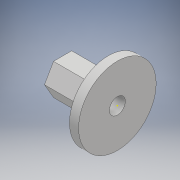
# Autodesk Inventor part: InnerLayerHub3mm
Saved by Autodesk Inventor 2018 (Build 220112000, 112)
## iProperties
Created: 2019-06-05
Part Number: InnerLayerHub3mm
Material: Generic
Document SubType Name: Modeling
Designer: Aditya Kendre
Density: 1 g/cm^3
Appearance: Default
Author: Aditya Kendre
Autodesk Inventor part; units mm, degrees
ref_plane "YZ Plane" through (0, 0, 0) normal (1, 0, 0) x (0, 1, 0)
ref_plane "XZ Plane" through (0, 0, 0) normal (0, 1, 0) x (-1, 0, 0)
ref_plane "XY Plane" through (0, 0, 0) normal (0, 0, 1) x (1, 0, 0)
sketch "Sketch1" plane through (0, 0, 0) normal (1, 0, 0) x (0, 1, 0)
  line L0 (2, 0) -> (-2, 0) construction
  line L1 (-2, 0) -> (-2, -15.7322) construction
  line L2 (-2, -15.7322) -> (2, -15.7322) construction
  line L3 (2, -15.7322) -> (2, 0) construction
  line L4 (2, -3.4446) -> (-1.9831, -3.4544)
  line L5 (-1.9831, -3.4544) -> (-3.9831, -0.0097)
  line L6 (-3.9831, -0.0097) -> (-2, 3.4446)
  line L7 (-2, 3.4446) -> (1.9831, 3.4544)
  line L8 (1.9831, 3.4544) -> (3.9831, 0.0097)
  line L9 (3.9831, 0.0097) -> (2, -3.4446)
  point P0 (0, 0)
  point P1 (0, 0)
  dimension "d0" = 4
  constraints: 20 end point, 2 parallel, 1 coincident, 1 horizontal, 1 perpendicular, 1 point on line, 13 other
  measures "d0" distance of L2.end L1.end
extrude "Extrusion1" add sketch "Sketch1" along normal blind 4 and the other way blind 6
sketch "Sketch2" plane through (4, 0, 0) normal (1, 0, 0) x (0, 0, -1)
  line L0 (3.4446, 2) -> (-0.0097, 3.9831) projected
  circle A0 centre (0, 0) radius 3.9832
  constraints: 1 coincident, 3 other
extrude "Extrusion2" add sketch "Sketch2" along normal blind 2
sketch "Sketch3" plane through (6, 0, 0) normal (1, 0, 0) x (0, 0, -1)
  point P0 (0, 0)
sketch "Sketch4" plane through (4, 0, 0) normal (-1, 0, 0) x (0, 0, 1)
  circle A0 centre (0, 0) radius 6
  dimension "d5" = 12
  constraints: 1 centre point, 1 coincident
  measures "d5" diameter of A0
extrude "Extrusion3" add sketch "Sketch4" against normal blind 2
sketch "Sketch5" plane through (6, 0, 0) normal (1, 0, 0) x (0, 0, -1)
  circle A0 centre (0, 0) radius 1.5
  dimension "d8" = 3
  constraints: 1 centre point, 1 coincident
  measures "d8" diameter of A0
extrude "Extrusion4" cut sketch "Sketch5" against normal blind 6
sketch "Sketch6" plane through (6, 0, 0) normal (1, 0, 0) x (0, 0, -1)
  point P0 (0, 0)
sketch "Sketch7" plane through (6, 0, 0) normal (1, 0, 0) x (0, 0, -1)
  circle A0 centre (0, 0) radius 8.5
  dimension "d11" = 17
  constraints: 1 centre point, 1 coincident
  measures "d11" diameter of A0
extrude "Extrusion5" add sketch "Sketch7" against normal blind 2
sketch "Sketch8" plane through (-6, 0, 0) normal (-1, 0, 0) x (0, 0, 1)
  circle A0 centre (0, 0) radius 1.75
  dimension "d16" = 3.5
  constraints: 1 centre point, 1 coincident
  measures "d16" diameter of A0
extrude "Extrusion6" cut sketch "Sketch8" against normal blind 12.25
body "Solid1"
